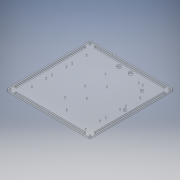
# Autodesk Inventor part: mid
Saved by Autodesk Inventor 2019 (Build 230136000, 136)
## iProperties
Created: 2018-04-27
Part Number: mid
Material: Polycarbonate, Clear
Document SubType Name: Modeling
Designer: Phil Erle
Density: 1.2 g/cm^3
Appearance: Polycarbonate - Clear
Author: Phil Erle
Autodesk Inventor part; units mm, degrees
ref_plane "YZ Plane" through (0, 0, 0) normal (1, 0, 0) x (0, 1, 0)
ref_plane "XZ Plane" through (0, 0, 0) normal (0, 1, 0) x (-1, 0, 0)
ref_plane "XY Plane" through (0, 0, 0) normal (0, 0, 1) x (1, 0, 0)
sketch "Sketch1" plane through (0, 0, 0) normal (0, 0, 1) x (1, 0, 0)
  line L0 (-145, -145) -> (145, -145)
  line L1 (145, -145) -> (145, 145)
  line L2 (145, 145) -> (-145, 145)
  line L3 (-145, 145) -> (-145, -145)
  line L4 (-145, -145) -> (145, 145) construction
  line L5 (145, -145) -> (-145, 145) construction
  point P0 (0, 0)
  dimension "d0" = 290
  dimension "d1" = 290
  constraints: 12 end point, 2 midpoint, 2 parallel, 1 horizontal, 1 perpendicular
  measures "d0" distance of L2.end L1.end
  measures "d1" distance of L1.end L0.end
extrude "Extrusion1" add sketch "Sketch1" along normal blind 5
sketch "Sketch2" plane through (0, 0, 5) normal (0, 0, 1) x (1, 0, 0)
  line L0 (-137.5, -137.5) -> (137.5, -137.5) construction
  line L1 (137.5, -137.5) -> (137.5, 137.5) construction
  line L2 (137.5, 137.5) -> (-137.5, 137.5) construction
  line L3 (-137.5, 137.5) -> (-137.5, -137.5) construction
  line L4 (-137.5, -137.5) -> (137.5, 137.5) construction
  line L5 (137.5, -137.5) -> (-137.5, 137.5) construction
  point P0 (0, 0)
  dimension "d4" = 275
  dimension "d5" = 275
  constraints: 12 end point, 4 coincident, 2 midpoint, 2 parallel, 1 horizontal, 1 perpendicular
  measures "d4" distance of L2.end L1.end
  measures "d5" distance of L1.end L0.end
hole "Hole1" at (-137.5, 137.5, 5) at (137.5, 137.5, 5) at (137.5, -137.5, 5) at (-137.5, -137.5, 5) direction (0, 0, -1) diameter 5.5 depth 8 tip angle 118 clearance for "Countersunk Flat Head Screw DIN EN ISO 2009" size "M5" standard "DIN"
fillet "Fillet1" radius 6 4 edges at (145, -145, 2.5) (-145, -145, 2.5) (145, 145, 2.5) (-145, 145, 2.5)
sketch "Sketch3" plane through (0, 0, 5) normal (0, 0, 1) x (1, 0, 0)
  line L0 (-110, -20.75) -> (-20, -20.75) construction
  line L1 (-20, -20.75) -> (-20, 28.75) construction
  line L2 (-20, 28.75) -> (-110, 28.75) construction
  line L3 (-110, 28.75) -> (-110, -20.75) construction
  line L4 (-139, -145) -> (139, -145) projected
  arc A0 (-139, 145) -> (-145, 139) centre (-139, 139) ccw projected
  line L5 (-145, 139) -> (-145, -139) projected
  arc A1 (-145, -139) -> (-139, -145) centre (-139, -139) ccw projected
  line L6 (-139, -145) -> (139, -145) projected
  arc A2 (139, -145) -> (145, -139) centre (139, -139) ccw projected
  line L7 (145, -139) -> (145, 139) projected
  arc A3 (145, 139) -> (139, 145) centre (139, 139) ccw projected
  line L8 (139, 145) -> (-139, 145) projected
  circle A4 centre (137.5, -137.5) radius 2.75 projected
  circle A5 centre (-137.5, 137.5) radius 2.75 projected
  circle A6 centre (137.5, 137.5) radius 2.75 projected
  circle A7 centre (-137.5, -137.5) radius 2.75 projected
  line L9 (-110, -90.25) -> (-20, -90.25) construction
  line L10 (-20, -90.25) -> (-20, -40.75) construction
  line L11 (-20, -40.75) -> (-110, -40.75) construction
  line L12 (-110, -40.75) -> (-110, -90.25) construction
  line L13 (20, -55.5) -> (110, -55.5) construction
  line L14 (110, -55.5) -> (110, -6) construction
  line L15 (110, -6) -> (20, -6) construction
  line L16 (20, -6) -> (20, -55.5) construction
  line L17 (-110, 48.75) -> (-20, 48.75) construction
  line L18 (-20, 48.75) -> (-20, 98.25) construction
  line L19 (-20, 98.25) -> (-110, 98.25) construction
  line L20 (-110, 98.25) -> (-110, 48.75) construction
  line L21 (20, -125) -> (110, -125) construction
  line L22 (110, -125) -> (110, -75.5) construction
  line L23 (110, -75.5) -> (20, -75.5) construction
  line L24 (20, -75.5) -> (20, -125) construction
  line L25 (20, 14) -> (110, 14) construction
  line L26 (110, 14) -> (110, 63.5) construction
  line L27 (110, 63.5) -> (20, 63.5) construction
  line L28 (20, 63.5) -> (20, 14) construction
  point P0 (0, 0)
  point P1 (-20, 73.5)
  point P2 (20, 38.75)
  point P3 (20, -30.75)
  point P4 (-20, -65.5)
  point P5 (20, -100.25)
  point P6 (-20, 4)
  dimension "d14" = 49.5
  dimension "d16" = 49.5
  dimension "d17" = 90
  dimension "d20" = 49.5
  dimension "d25" = 90
  dimension "d26" = 290
  dimension "d29" = 20
  dimension "d71" = 49.5
  dimension "d72" = 49.5
  dimension "d73" = 49.5
  dimension "d75" = 20
  dimension "d76" = 20
  dimension "d77" = 20
  dimension "d78" = 54.75
  dimension "d79" = 20
  dimension "d81" = 40
  dimension "d82" = 35
  constraints: 48 end point, 24 coincident, 12 parallel, 8 vertical alignment, 6 horizontal, 6 midpoint, 6 perpendicular
  measures "d14" distance of L2.end L0.start
  measures "d16" distance of L11.end L9.start
  measures "d17" distance of L10.end L11.end
  measures "d20" distance of L19.end L17.start
  measures "d25" distance of L26.end L27.end
  measures "d26" distance between parallel lines of L7 L5
  measures "d29" distance of point (-110, 48.75) point (-110, 28.75)
  measures "d71" distance of point (110, -6) point (110, -55.5)
  measures "d72" distance of point (110, -125) point (110, -75.5)
  measures "d73" distance of point (110, 63.5) point (110, 14)
  measures "d75" distance from line of L4 point (110, -125)
  measures "d76" distance of point (110, -55.5) point (110, -75.5)
  measures "d77" distance of L26.start point (110, -6)
  measures "d78" distance between parallel lines of L4 L9
  measures "d79" distance between parallel lines of L11 L0
  measures "d81" horizontal distance of point (20, -75.5) point (-20, -90.25)
  measures "d82" distance from line of L5 L9.start
hole "Hole2" at (-20, 73.5, 5) at (20, 38.75, 5) at (20, -30.75, 5) at (-20, -65.5, 5) at (20, -100.25, 5) at (110, 63.5, 5) at (110, 14, 5) at (110, -6, 5) at (110, -55.5, 5) at (110, -75.5, 5) at (110, -125, 5) at (-110, -40.75, 5) at (-110, -90.25, 5) at (-110, -20.75, 5) at (-110, 28.75, 5) at (-110, 48.75, 5) at (-110, 98.25, 5) at (-20, 4, 5) direction (0, 0, -1) diameter 3.4 end through all clearance for "Countersunk Flat Head Screw DIN EN ISO 2009" size "M3" standard "DIN"
sketch "Sketch4" plane through (0, 0, 5) normal (0, 0, 1) x (1, 0, 0)
  line L0 (-120, -140) -> (120, -140)
  line L1 (120, -140) -> (120, -135)
  line L2 (120, -135) -> (-120, -135)
  line L3 (-120, -135) -> (-120, -140)
  line L4 (140, -120) -> (135, -120)
  line L5 (135, -120) -> (135, 120)
  line L6 (135, 120) -> (140, 120)
  line L7 (140, 120) -> (140, -120)
  line L8 (120, 140) -> (-120, 140)
  line L9 (-120, 140) -> (-120, 135)
  line L10 (-120, 135) -> (120, 135)
  line L11 (120, 135) -> (120, 140)
  line L12 (-135, 120) -> (-140, 120)
  line L13 (-140, 120) -> (-140, -120)
  line L14 (-140, -120) -> (-135, -120)
  line L15 (-135, -120) -> (-135, 120)
  line L16 (-139, -145) -> (139, -145) projected
  line L17 (-145, 139) -> (-145, -139) projected
  line L18 (139, 145) -> (-139, 145) projected
  line L19 (145, -139) -> (145, 139) projected
  point P0 (0, 0)
  point P1 (0, -140)
  point P2 (-140, 0)
  point P3 (140, 0)
  point P4 (0, 140)
  dimension "d39" = 5
  dimension "d40" = 5
  dimension "d41" = 5
  dimension "d42" = 5
  dimension "d43" = 240
  dimension "d44" = 240
  dimension "d45" = 240
  dimension "d46" = 5
  dimension "d47" = 5
  dimension "d48" = 5
  dimension "d49" = 5
  constraints: 32 end point, 8 parallel, 4 horizontal, 4 midpoint, 4 perpendicular, 2 horizontal alignment, 2 vertical alignment, 1 point on line
  measures "d39" distance of L2.end L0.start
  measures "d40" distance of L13.end L14.end
  measures "d41" distance of L4.start L4.end
  measures "d42" distance of L10.end L8.start
  measures "d43" distance of L0.start L0.end
  measures "d44" distance of L12.end L13.end
  measures "d45" distance of L6.end L4.start
  measures "d46" distance between parallel lines of L16 L0
  measures "d47" distance between parallel lines of L17 L13
  measures "d48" distance between parallel lines of L18 L8
  measures "d49" distance between parallel lines of L19 L7
extrude "Extrusion2" cut sketch "Sketch4" against normal through all
sketch "Sketch5" plane through (0, 0, 5) normal (0, 0, 1) x (1, 0, 0)
  point P0 (0, 0)
  point P1 (120, 0)
  dimension "d60" = 120
  constraints: 1 horizontal alignment
  measures "d60" distance of point (0, 0) point (120, 0)
hole "Hole3" at (120, 0, 5) direction (0, 0, -1) diameter 8 depth 8 tip angle 118
sketch "Sketch6" plane through (0, 0, 5) normal (0, 0, 1) x (1, 0, 0)
  line L0 (-20, 120) -> (20, 120) construction
  point P0 (0, 0)
  point P1 (0, 120)
  dimension "d61" = 40
  dimension "d70" = 120
  constraints: 2 coincident, 2 end point, 1 horizontal, 1 midpoint, 1 vertical alignment
  measures "d61" distance of L0.start L0.end
  measures "d70" distance of point (0, 120) point (0, 0)
hole "Hole4" at (-20, 120, 5) at (20, 120, 5) direction (0, 0, -1) diameter 12 depth 8 tip angle 118
sketch "Sketch7" plane through (0, 0, 5) normal (0, 0, 1) x (1, 0, 0)
  line L0 (77, 105) -> (63, 105) construction
  point P0 (0, 0)
  dimension "d83" = 14
  dimension "d84" = 105
  dimension "d85" = 63
  constraints: 2 coincident, 2 end point, 1 horizontal
  measures "d83" distance of L0.start L0.end
  measures "d84" vertical distance of point (0, 0) point (77, 105)
  measures "d85" horizontal distance of point (0, 0) point (63, 105)
hole "Hole5" at (77, 105, 5) at (63, 105, 5) direction (0, 0, -1) diameter 3.4 depth 8 tip angle 118 clearance for "Countersunk Flat Head Screw DIN EN ISO 2009" size "M3" standard "DIN"
sketch "Sketch8" plane through (0, 0, 5) normal (0, 0, 1) x (1, 0, 0)
  circle A0 centre (77, 105) radius 1.7 projected
  point P0 (0, 0)
  point P1 (92, 87)
  dimension "d93" = 15
  dimension "d94" = 18
  measures "d93" horizontal distance of A0.centre point (92, 87)
  measures "d94" vertical distance of point (92, 87) A0.centre
hole "Hole6" at (92, 87, 5) direction (0, 0, -1) diameter 8 depth 8 tip angle 118
equation "\"d29\" = d28"
equation "\"d76\" = d28"
equation "\"d77\" = d28"
equation "\"d28\" = 20"
body "Solid1"
